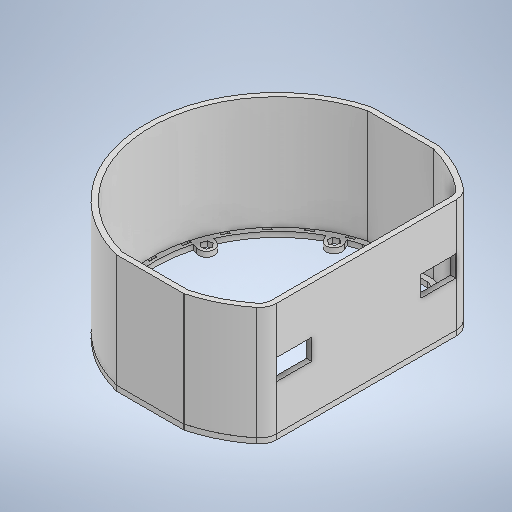
# Autodesk Inventor part: carcasa
Saved by Autodesk Inventor 2025.2 (Build 292293000, 293)
## iProperties
Created: 2025-08-27
Part Number: carcasa
Material: Generic
Document SubType Name: Modeling
Designer: cdavi
Density: 1 g/cm^3
Appearance: Default
Author: cdavi
Autodesk Inventor part; units mm, degrees
ref_plane "YZ Plane" through (0, 0, 0) normal (1, 0, 0) x (0, 1, 0)
ref_plane "XZ Plane" through (0, 0, 0) normal (0, 1, 0) x (-1, 0, 0)
ref_plane "XY Plane" through (0, 0, 0) normal (0, 0, 1) x (1, 0, 0)
sketch "Sketch1" plane through (0, 0, 0) normal (0, 1, 0) x (-1, 0, 0)
  line L0 (18.2688, 67.5) -> (-18.2688, 67.5)
  line L1 (0, 0) -> (-51, 0) construction
  line L2 (19.0722, 73.5) -> (-19.0722, 73.5)
  line L3 (18.2688, -67.5) -> (-18.5405, -67.5)
  line L4 (19.0722, -73.5) -> (-19.0722, -73.5)
  line L5 (0, 0) -> (0, 73.5) construction
  line L6 (-45, 48.734) -> (-45, -48.734)
  line L7 (-51, 51.7204) -> (-51, -51.7204)
  arc A0 (-40.8333, -56.8563) -> (-18.5405, -67.5) centre (0, 0) ccw
  arc A1 (-47.2121, -59.5568) -> (-19.5877, -73.4324) centre (0, 0) ccw
  arc A2 (19.5877, -73.4324) -> (19.5877, 73.4324) centre (0, 0) ccw
  arc A3 (-19.5877, 73.4324) -> (-47.2121, 59.5568) centre (0, 0) ccw
  arc A4 (18.8061, -67.4265) -> (18.8061, 67.4265) centre (0, 0) ccw
  arc A5 (-18.8061, 67.4265) -> (-40.8333, 56.8563) centre (0, 0) ccw
  arc A6 (-19.5877, -73.4324) -> (-19.0722, -73.5) centre (-19.0722, -71.5) ccw
  arc A7 (19.0722, -73.5) -> (19.5877, -73.4324) centre (19.0722, -71.5) ccw
  arc A8 (18.2688, -67.5) -> (18.8061, -67.4265) centre (18.2688, -65.5) ccw
  arc A9 (18.8061, 67.4265) -> (18.2688, 67.5) centre (18.2688, 65.5) ccw
  arc A10 (19.5877, 73.4324) -> (19.0722, 73.5) centre (19.0722, 71.5) ccw
  arc A11 (-18.2688, 67.5) -> (-18.8061, 67.4265) centre (-18.2688, 65.5) ccw
  arc A12 (-19.0722, 73.5) -> (-19.5877, 73.4324) centre (-19.0722, 71.5) ccw
  arc A13 (-40.8333, 56.8563) -> (-45, 48.734) centre (-35, 48.734) ccw
  arc A14 (-47.2121, 59.5568) -> (-51, 51.7204) centre (-41, 51.7204) ccw
  arc A15 (-51, -51.7204) -> (-47.2121, -59.5568) centre (-41, -51.7204) ccw
  arc A16 (-45, -48.734) -> (-40.8333, -56.8563) centre (-35, -48.734) ccw
  line L8 (18.9407, 70.5) -> (-18.9407, 70.5)
  arc A17 (-18.9407, 70.5) -> (-45.3485, 57.2059) centre (0, 0) ccw
  arc A18 (-45.3485, 57.2059) -> (-48, 51.7204) centre (-41, 51.7204) ccw
  line L9 (-48, 51.7204) -> (-48, -51.7204)
  arc A19 (-48, -51.7204) -> (-45.3485, -57.2059) centre (-41, -51.7204) ccw
  arc A20 (-45.3485, -57.2059) -> (-18.9407, -70.5) centre (0, 0) ccw
  line L10 (-18.9407, -70.5) -> (18.9407, -70.5)
  arc A21 (18.9407, -70.5) -> (18.9407, 70.5) centre (0, 0) ccw
  line L11 (18.9407, 70.5) -> (0, 0) construction
  line L12 (0, 0) -> (18.9407, -70.5) construction
  line L13 (0, 0) -> (-18.9407, -70.5) construction
  point P0 (-19.3326, 73.5)
  point P1 (18.5405, -67.5)
  point P2 (19.3326, -73.5)
  point P3 (-19.3326, -73.5)
  point P4 (-51, -56.3471)
  point P5 (-45, 53.619)
  point P6 (-45, -53.619)
  point P7 (-51, 56.3471)
  point P8 (19.3326, 73.5)
  point P9 (18.5405, 67.5)
  point P10 (-18.5405, 67.5)
  dimension "d2" = 67.5
  dimension "d4" = 6
  dimension "d6" = 45
  dimension "d7" = 6
  dimension "d8" = 2
  dimension "d9" = 10
  dimension "d10" = 70
  dimension "d11" = 76
  dimension "d12" = 70
  dimension "d13" = 76
  dimension "d185" = 3
  constraints: 55 point on circle, 28 end point, 22 centre point, 22 tangent, 11 point on line, 9 equal radius, 4 symmetric about line, 3 vertical, 2 coincident, 2 horizontal, 2 midpoint, 1 parallel, 7 other
  measures "d2" distance between parallel lines of L1 L0
  measures "d4" distance between parallel lines of L0 L2
  measures "d6" distance between parallel lines of L6 L5
  measures "d7" distance between parallel lines of L7 L6
  measures "d8" radius of A6
  measures "d9" radius of A13
  measures "d10" radius of A4
  measures "d11" radius of A2
  measures "d12" radius of A0
  measures "d13" radius of A1
  measures "d185" radial gap between concentric circles of A2 A21
extrude "Extrusion1" add sketch "Sketch1" along normal blind 65 contours A10 A2 A7 L4 A6 A1 A15 L7 A14 A3 A12 L2
sketch "Sketch2" plane through (51, 0, 51.7204) normal (1, 0, 0) x (0, 0, -1)
  line L0 (51.7204, 0) -> (51.7204, 67.372) construction
  line L1 (0.288, 38) -> (20.288, 38)
  line L2 (20.288, 38) -> (20.288, 26)
  line L3 (20.288, 26) -> (0.288, 26)
  line L4 (0.288, 26) -> (0.288, 38)
  line L5 (0, 0) -> (103.4408, 0) projected
  line L6 (-21.712, 0) -> (-21.712, 65) projected
  line L7 (103.1528, 38) -> (83.1528, 38)
  line L8 (83.1528, 38) -> (83.1528, 26)
  line L9 (83.1528, 26) -> (103.1528, 26)
  line L10 (103.1528, 26) -> (103.1528, 38)
  dimension "d16" = 26
  dimension "d17" = 22
  dimension "d18" = 12
  dimension "d19" = 20
  constraints: 18 end point, 4 symmetric about line, 2 parallel, 1 horizontal, 1 perpendicular, 1 vertical
  measures "d16" distance between parallel lines of L5 L3
  measures "d17" distance between parallel lines of L4 L6
  measures "d18" distance of L1.end L2.end
  measures "d19" distance of L1.start L1.end
extrude "Extrusion2" cut sketch "Sketch2" against normal blind 7
extrude "Extrusion4" add sketch "Sketch1" along normal blind 3 from surface at 65 separate body contours A9 A4 A8 L3 A0 A16 L6 A13 A5 A11 L0 | A10 A2 A7 L4 A6 A1 A15 L7 A14 A3 A12 L2 | A21 L10 A20 A19 L9 A18 A17 L8
sketch "Sketch5" plane through (-19.0722, 68, 73.5) normal (0, 1, 0) x (1, 0, 0)
  circle A0 centre (19.0722, 73.5) radius 8.5
  circle A1 centre (-10.9278, 73.5) radius 2.5
  line L0 (27.1963, 71) -> (36.0722, 71)
  line L1 (36.0722, 71) -> (36.0722, 76)
  line L2 (36.0722, 76) -> (27.1963, 76)
  point P0 (36.0722, 73.5)
  dimension "d26" = 17
  dimension "d27" = 5
  dimension "d31" = 5
  dimension "d32" = 17
  dimension "d47" = 30
  constraints: 6 end point, 2 centre point, 2 horizontal alignment, 2 perpendicular, 2 point on circle, 1 coincident, 1 horizontal, 1 midpoint
  measures "d26" diameter of A0
  measures "d27" diameter of A1
  measures "d31" distance between parallel lines of L2 L0
  measures "d32" distance from line of A0.centre L1
  measures "d47" distance of A0.centre A1.centre
extrude "Extrusion5" cut sketch "Sketch5" against normal through all bodies 2
sketch "Sketch6" plane through (0, 0, 0) normal (0, 1, 0) x (-1, 0, 0)
  circle A0 centre (0, 0) radius 67 construction
  line L0 (19.0722, 73.5) -> (-19.0722, 73.5) projected
  arc A1 (-19.5877, 73.4324) -> (-47.2121, 59.5568) centre (0, 0) ccw projected
  arc A2 (-47.2121, 59.5568) -> (-51, 51.7204) centre (-41, 51.7204) ccw projected
  line L1 (-51, 51.7204) -> (-51, -51.7204) projected
  arc A3 (-51, -51.7204) -> (-47.2121, -59.5568) centre (-41, -51.7204) ccw projected
  arc A4 (-47.2121, -59.5568) -> (-19.5877, -73.4324) centre (0, 0) ccw projected
  line L2 (-19.0722, -73.5) -> (19.0722, -73.5) projected
  arc A5 (19.5877, -73.4324) -> (19.5877, 73.4324) centre (0, 0) ccw projected
  line L3 (0, 0) -> (63.1919, 22.2662) construction
  line L4 (0, 0) -> (76, 0) construction
  circle A6 centre (63.1919, 22.2662) radius 2.95 construction
  line L5 (0, 0) -> (0, -67) construction
  circle A7 centre (28.3154, 60.7226) radius 2.95 construction
  line L6 (28.3154, 60.7226) -> (0, 0) construction
  circle A8 centre (-41.5, 20) radius 2.95 construction
  circle A9 centre (-28.3154, 60.7226) radius 2.95 construction
  line L7 (-28.3154, 60.7226) -> (0, 0) construction
  arc A10 (-19.5877, -73.4324) -> (-19.0722, -73.5) centre (-19.0722, -71.5) ccw projected
  arc A11 (19.0722, -73.5) -> (19.5877, -73.4324) centre (19.0722, -71.5) ccw projected
  arc A12 (19.5877, 73.4324) -> (19.0722, 73.5) centre (19.0722, 71.5) ccw projected
  arc A13 (-19.0722, 73.5) -> (-19.5877, 73.4324) centre (-19.0722, 71.5) ccw projected
  circle A14 centre (63.1919, -22.2662) radius 2.95 construction
  circle A15 centre (28.3154, -60.7226) radius 2.95 construction
  circle A16 centre (-41.5, -20) radius 2.95 construction
  circle A17 centre (-28.3154, -60.7226) radius 2.95 construction
  arc A18 (61.5547, 26.4578) -> (64.544, 17.9741) centre (63.1919, 22.2662) ccw
  arc A19 (24.1755, 62.4864) -> (32.3276, 58.685) centre (28.3154, 60.7226) ccw
  line L8 (60.2922, 22.8083) -> (62.2115, 25.0485)
  line L9 (62.2115, 25.0485) -> (65.1113, 24.5064)
  line L10 (65.1113, 24.5064) -> (66.0917, 21.724)
  line L11 (66.0917, 21.724) -> (64.1723, 19.4838)
  line L12 (64.1723, 19.4838) -> (61.2725, 20.026)
  line L13 (61.2725, 20.026) -> (60.2922, 22.8083)
  line L14 (25.8989, 59.0306) -> (25.6418, 61.9693)
  line L15 (25.6418, 61.9693) -> (28.0583, 63.6614)
  line L16 (28.0583, 63.6614) -> (30.7319, 62.4147)
  line L17 (30.7319, 62.4147) -> (30.989, 59.4759)
  line L18 (30.989, 59.4759) -> (28.5725, 57.7838)
  line L19 (28.5725, 57.7838) -> (25.8989, 59.0306)
  arc A20 (-41.5, 15.5) -> (-41.5, 24.5) centre (-41.5, 20) ccw
  line L20 (-44.0548, 18.525) -> (-44.0548, 21.475)
  line L21 (-44.0548, 21.475) -> (-41.5, 22.95)
  line L22 (-41.5, 22.95) -> (-38.9452, 21.475)
  line L23 (-38.9452, 21.475) -> (-38.9452, 18.525)
  line L24 (-38.9452, 18.525) -> (-41.5, 17.05)
  line L25 (-41.5, 17.05) -> (-44.0548, 18.525)
  line L26 (-41.5, 24.5) -> (-45, 24.5)
  line L27 (-41.5, 15.5) -> (-45, 15.5)
  arc A21 (-32.3276, 58.685) -> (-24.1755, 62.4864) centre (-28.3154, 60.7226) ccw
  line L28 (-28.5725, 57.7838) -> (-30.989, 59.4759)
  line L29 (-30.989, 59.4759) -> (-30.7319, 62.4147)
  line L30 (-30.7319, 62.4147) -> (-28.0583, 63.6614)
  line L31 (-28.0583, 63.6614) -> (-25.6418, 61.9693)
  line L32 (-25.6418, 61.9693) -> (-25.8989, 59.0306)
  line L33 (-25.8989, 59.0306) -> (-28.5725, 57.7838)
  line L34 (-32.3276, 58.685) -> (-33.6868, 61.3612)
  arc A22 (64.544, -17.9741) -> (61.5547, -26.4578) centre (63.1919, -22.2662) ccw
  arc A23 (32.3276, -58.685) -> (24.1755, -62.4864) centre (28.3154, -60.7226) ccw
  arc A24 (-41.5, -24.5) -> (-41.5, -15.5) centre (-41.5, -20) ccw
  line L35 (-41.5, -24.5) -> (-45, -24.5)
  line L36 (-41.5, -15.5) -> (-45, -15.5)
  arc A25 (-24.1755, -62.4864) -> (-32.3276, -58.685) centre (-28.3154, -60.7226) ccw
  line L37 (-32.3276, -58.685) -> (-33.6868, -61.3612)
  line L38 (60.2922, -22.8083) -> (62.2115, -25.0485)
  line L39 (62.2115, -25.0485) -> (65.1113, -24.5064)
  line L40 (65.1113, -24.5064) -> (66.0917, -21.724)
  line L41 (66.0917, -21.724) -> (64.1723, -19.4838)
  line L42 (64.1723, -19.4838) -> (61.2725, -20.026)
  line L43 (61.2725, -20.026) -> (60.2922, -22.8083)
  line L44 (25.8989, -59.0306) -> (25.6418, -61.9693)
  line L45 (25.6418, -61.9693) -> (28.0583, -63.6614)
  line L46 (28.0583, -63.6614) -> (30.7319, -62.4147)
  line L47 (30.7319, -62.4147) -> (30.989, -59.4759)
  line L48 (30.989, -59.4759) -> (28.5725, -57.7838)
  line L49 (28.5725, -57.7838) -> (25.8989, -59.0306)
  line L50 (-28.5725, -57.7838) -> (-30.989, -59.4759)
  line L51 (-30.989, -59.4759) -> (-30.7319, -62.4147)
  line L52 (-30.7319, -62.4147) -> (-28.0583, -63.6614)
  line L53 (-28.0583, -63.6614) -> (-25.6418, -61.9693)
  line L54 (-25.6418, -61.9693) -> (-25.8989, -59.0306)
  line L55 (-25.8989, -59.0306) -> (-28.5725, -57.7838)
  line L56 (-44.0548, -18.525) -> (-44.0548, -21.475)
  line L57 (-44.0548, -21.475) -> (-41.5, -22.95)
  line L58 (-41.5, -22.95) -> (-38.9452, -21.475)
  line L59 (-38.9452, -21.475) -> (-38.9452, -18.525)
  line L60 (-38.9452, -18.525) -> (-41.5, -17.05)
  line L61 (-41.5, -17.05) -> (-44.0548, -18.525)
  line L62 (61.5547, 26.4578) -> (64.3507, 27.5498)
  line L63 (64.544, 17.9741) -> (67.4069, 18.876)
  line L64 (32.3276, 58.685) -> (33.6868, 61.3612)
  line L65 (61.5547, -26.4578) -> (64.3507, -27.5498)
  line L66 (64.544, -17.9741) -> (67.4069, -18.876)
  line L67 (32.3276, -58.685) -> (33.6868, -61.3612)
  line L68 (-24.1755, 62.4864) -> (-25.3519, 65.2478)
  line L69 (24.1755, 62.4864) -> (25.3519, 65.2478)
  line L70 (-24.1755, -62.4864) -> (-25.3519, -65.2478)
  line L71 (24.1755, -62.4864) -> (25.3519, -65.2478)
  arc A26 (-18.5405, 67.5) -> (-43.4848, 54.855) centre (0, 0) ccw
  line L72 (-18.5405, 67.5) -> (18.5405, 67.5)
  arc A27 (18.5405, -67.5) -> (18.5405, 67.5) centre (0, 0) ccw
  line L73 (18.5405, -67.5) -> (-18.5405, -67.5)
  arc A28 (-43.4848, -54.855) -> (-18.5405, -67.5) centre (0, 0) ccw
  arc A29 (-45, -51.7204) -> (-43.4848, -54.855) centre (-41, -51.7204) ccw
  line L74 (-45, -51.7204) -> (-45, 51.7204)
  arc A30 (-43.4848, 54.855) -> (-45, 51.7204) centre (-41, 51.7204) ccw
  point P0 (28.3154, 60.7226)
  point P1 (28.3154, 60.7226)
  point P2 (61.5547, -26.4578)
  point P3 (32.3276, -58.685)
  point P4 (-24.1755, -62.4864)
  dimension "d33" = 134
  dimension "d39" = 5.9
  dimension "d37" = 19.41
  dimension "d38" = 25
  dimension "d40" = 20
  dimension "d42" = 25
  dimension "d61" = 9
  dimension "d62" = 9
  dimension "d63" = 9
  dimension "d64" = 9
  dimension "d186" = 6
  dimension "d187" = 3.5
  constraints: 144 end point, 48 symmetric about line, 27 point on circle, 17 centre point, 10 coincident, 8 tangent, 4 perpendicular, 3 horizontal, 2 point on line, 1 vertical, 93 other
  measures "d37" angle of L4 L3
  measures "d38" angle of L5 L6
  measures "d40" distance from line of point (-41.5, 20) L4
  measures "d42" angle of L5 L7
  measures "d61" diameter of A18
  measures "d62" diameter of A19
  measures "d63" diameter of A20
  measures "d64" diameter of A21
  measures "d186" radial gap between concentric circles of A1 A26
  measures "d187" distance from line of L74 A20.centre
extrude "Extrusion6" add sketch "Sketch6" against normal blind 3 separate body contours A12 A5 A11 L2 A10 A4 A3 L1 A2 A1 A13 L0 | L62 A27 L63 A18 | L64 A19 L69 A27 | A27 L65 A22 L66 | A27 L71 A23 L67 | L68 A21 L34 A26 | A28 L37 A25 L70 | L26 A20 L27 L74 | L36 A24 L35 L74
sketch "Sketch8" plane through (0, 0, 0) normal (0, 1, 0) x (1, 0, 0)
  arc A0 (-19.5877, 73.4324) -> (-19.5877, -73.4324) centre (0, 0) ccw projected
  line L0 (-76, 0) -> (-70, 0)
  line L1 (-73, 0) -> (-73, -2)
  line L2 (-73, 0) -> (-73, 2)
  line L3 (-73, 2) -> (-71.5, 2)
  line L4 (-71.5, 2) -> (-71.5, -2)
  line L5 (-71.5, -2) -> (-74.5, -2)
  line L6 (-74.5, -2) -> (-74.5, 2)
  line L7 (-74.5, 2) -> (-71.5, 2)
  line L8 (-69.901, -15.1692) -> (-68.9437, -19.053)
  line L9 (-68.9437, -19.053) -> (-71.8565, -19.7709)
  line L10 (-71.8565, -19.7709) -> (-72.8138, -15.8871)
  line L11 (-71.3574, -15.5282) -> (-69.901, -15.1692)
  line L12 (-72.8138, -15.8871) -> (-69.901, -15.1692)
  line L13 (-64.2396, -31.4568) -> (-62.3807, -34.9986)
  line L14 (-62.3807, -34.9986) -> (-65.037, -36.3928)
  line L15 (-65.037, -36.3928) -> (-66.8959, -32.851)
  line L16 (-65.5677, -32.1539) -> (-64.2396, -31.4568)
  line L17 (-66.8959, -32.851) -> (-64.2396, -31.4568)
  line L18 (-54.8448, -45.9162) -> (-52.1923, -48.9103)
  line L19 (-52.1923, -48.9103) -> (-54.4378, -50.8997)
  line L20 (-54.4378, -50.8997) -> (-57.0903, -47.9056)
  line L21 (-55.9675, -46.9109) -> (-54.8448, -45.9162)
  line L22 (-57.0903, -47.9056) -> (-54.8448, -45.9162)
  line L23 (-42.2626, -57.7072) -> (-38.9707, -59.9795)
  line L24 (-38.9707, -59.9795) -> (-40.6749, -62.4484)
  line L25 (-40.6749, -62.4484) -> (-43.9668, -60.1762)
  line L26 (-43.1147, -58.9417) -> (-42.2626, -57.7072)
  line L27 (-43.9668, -60.1762) -> (-42.2626, -57.7072)
  line L28 (-27.2243, -66.1445) -> (-23.4842, -67.5629)
  line L29 (-23.4842, -67.5629) -> (-24.548, -70.3679)
  line L30 (-24.548, -70.3679) -> (-28.2881, -68.9495)
  line L31 (-27.7562, -67.547) -> (-27.2243, -66.1445)
  line L32 (-28.2881, -68.9495) -> (-27.2243, -66.1445)
  line L33 (-10.6038, -70.7376) -> (-6.633, -71.2198)
  line L34 (-6.633, -71.2198) -> (-6.9946, -74.1979)
  line L35 (-6.9946, -74.1979) -> (-10.9654, -73.7157)
  line L36 (-10.7846, -72.2267) -> (-10.6038, -70.7376)
  line L37 (-10.9654, -73.7157) -> (-10.6038, -70.7376)
  line L38 (6.633, -71.2198) -> (10.6038, -70.7376)
  line L39 (10.6038, -70.7376) -> (10.9654, -73.7157)
  line L40 (10.9654, -73.7157) -> (6.9946, -74.1979)
  line L41 (6.8138, -72.7088) -> (6.633, -71.2198)
  line L42 (6.9946, -74.1979) -> (6.633, -71.2198)
  line L43 (23.4842, -67.5629) -> (27.2243, -66.1445)
  line L44 (27.2243, -66.1445) -> (28.2881, -68.9495)
  line L45 (28.2881, -68.9495) -> (24.548, -70.3679)
  line L46 (24.0161, -68.9654) -> (23.4842, -67.5629)
  line L47 (24.548, -70.3679) -> (23.4842, -67.5629)
  line L48 (38.9707, -59.9795) -> (42.2626, -57.7072)
  line L49 (42.2626, -57.7072) -> (43.9668, -60.1762)
  line L50 (43.9668, -60.1762) -> (40.6749, -62.4484)
  line L51 (39.8228, -61.214) -> (38.9707, -59.9795)
  line L52 (40.6749, -62.4484) -> (38.9707, -59.9795)
  line L53 (52.1923, -48.9103) -> (54.8448, -45.9162)
  line L54 (54.8448, -45.9162) -> (57.0903, -47.9056)
  line L55 (57.0903, -47.9056) -> (54.4378, -50.8997)
  line L56 (53.315, -49.905) -> (52.1923, -48.9103)
  line L57 (54.4378, -50.8997) -> (52.1923, -48.9103)
  line L58 (62.3807, -34.9986) -> (64.2396, -31.4568)
  line L59 (64.2396, -31.4568) -> (66.8959, -32.851)
  line L60 (66.8959, -32.851) -> (65.037, -36.3928)
  line L61 (63.7088, -35.6957) -> (62.3807, -34.9986)
  line L62 (65.037, -36.3928) -> (62.3807, -34.9986)
  line L63 (68.9437, -19.053) -> (69.901, -15.1692)
  line L64 (69.901, -15.1692) -> (72.8138, -15.8871)
  line L65 (72.8138, -15.8871) -> (71.8565, -19.7709)
  line L66 (70.4001, -19.4119) -> (68.9437, -19.053)
  line L67 (71.8565, -19.7709) -> (68.9437, -19.053)
  line L68 (71.5, -2) -> (71.5, 2)
  line L69 (71.5, 2) -> (74.5, 2)
  line L70 (74.5, 2) -> (74.5, -2)
  line L71 (73, -2) -> (71.5, -2)
  line L72 (74.5, -2) -> (71.5, -2)
  line L73 (69.901, 15.1692) -> (68.9437, 19.053)
  line L74 (68.9437, 19.053) -> (71.8565, 19.7709)
  line L75 (71.8565, 19.7709) -> (72.8138, 15.8871)
  line L76 (71.3574, 15.5282) -> (69.901, 15.1692)
  line L77 (72.8138, 15.8871) -> (69.901, 15.1692)
  line L78 (64.2396, 31.4568) -> (62.3807, 34.9986)
  line L79 (62.3807, 34.9986) -> (65.037, 36.3928)
  line L80 (65.037, 36.3928) -> (66.8959, 32.851)
  line L81 (65.5677, 32.1539) -> (64.2396, 31.4568)
  line L82 (66.8959, 32.851) -> (64.2396, 31.4568)
  line L83 (54.8448, 45.9162) -> (52.1923, 48.9103)
  line L84 (52.1923, 48.9103) -> (54.4378, 50.8997)
  line L85 (54.4378, 50.8997) -> (57.0903, 47.9056)
  line L86 (55.9675, 46.9109) -> (54.8448, 45.9162)
  line L87 (57.0903, 47.9056) -> (54.8448, 45.9162)
  line L88 (42.2626, 57.7072) -> (38.9707, 59.9795)
  line L89 (38.9707, 59.9795) -> (40.6749, 62.4484)
  line L90 (40.6749, 62.4484) -> (43.9668, 60.1762)
  line L91 (43.1147, 58.9417) -> (42.2626, 57.7072)
  line L92 (43.9668, 60.1762) -> (42.2626, 57.7072)
  line L93 (27.2243, 66.1445) -> (23.4842, 67.5629)
  line L94 (23.4842, 67.5629) -> (24.548, 70.3679)
  line L95 (24.548, 70.3679) -> (28.2881, 68.9495)
  line L96 (27.7562, 67.547) -> (27.2243, 66.1445)
  line L97 (28.2881, 68.9495) -> (27.2243, 66.1445)
  line L98 (10.6038, 70.7376) -> (6.633, 71.2198)
  line L99 (6.633, 71.2198) -> (6.9946, 74.1979)
  line L100 (6.9946, 74.1979) -> (10.9654, 73.7157)
  line L101 (10.7846, 72.2267) -> (10.6038, 70.7376)
  line L102 (10.9654, 73.7157) -> (10.6038, 70.7376)
  line L103 (-6.633, 71.2198) -> (-10.6038, 70.7376)
  line L104 (-10.6038, 70.7376) -> (-10.9654, 73.7157)
  line L105 (-10.9654, 73.7157) -> (-6.9946, 74.1979)
  line L106 (-6.8138, 72.7088) -> (-6.633, 71.2198)
  line L107 (-6.9946, 74.1979) -> (-6.633, 71.2198)
  line L108 (-23.4842, 67.5629) -> (-27.2243, 66.1445)
  line L109 (-27.2243, 66.1445) -> (-28.2881, 68.9495)
  line L110 (-28.2881, 68.9495) -> (-24.548, 70.3679)
  line L111 (-24.0161, 68.9654) -> (-23.4842, 67.5629)
  line L112 (-24.548, 70.3679) -> (-23.4842, 67.5629)
  line L113 (-38.9707, 59.9795) -> (-42.2626, 57.7072)
  line L114 (-42.2626, 57.7072) -> (-43.9668, 60.1762)
  line L115 (-43.9668, 60.1762) -> (-40.6749, 62.4484)
  line L116 (-39.8228, 61.214) -> (-38.9707, 59.9795)
  line L117 (-40.6749, 62.4484) -> (-38.9707, 59.9795)
  line L118 (-52.1923, 48.9103) -> (-54.8448, 45.9162)
  line L119 (-54.8448, 45.9162) -> (-57.0903, 47.9056)
  line L120 (-57.0903, 47.9056) -> (-54.4378, 50.8997)
  line L121 (-53.315, 49.905) -> (-52.1923, 48.9103)
  line L122 (-54.4378, 50.8997) -> (-52.1923, 48.9103)
  line L123 (-62.3807, 34.9986) -> (-64.2396, 31.4568)
  line L124 (-64.2396, 31.4568) -> (-66.8959, 32.851)
  line L125 (-66.8959, 32.851) -> (-65.037, 36.3928)
  line L126 (-63.7088, 35.6957) -> (-62.3807, 34.9986)
  line L127 (-65.037, 36.3928) -> (-62.3807, 34.9986)
  line L128 (-68.9437, 19.053) -> (-69.901, 15.1692)
  line L129 (-69.901, 15.1692) -> (-72.8138, 15.8871)
  line L130 (-72.8138, 15.8871) -> (-71.8565, 19.7709)
  line L131 (-70.4001, 19.4119) -> (-68.9437, 19.053)
  line L132 (-71.8565, 19.7709) -> (-68.9437, 19.053)
  arc A1 (-67.4069, 18.876) -> (-67.4069, -18.876) centre (0, 0) ccw projected
  point P0 (-73, 2)
  dimension "d132" = 2
  dimension "d133" = 2
  dimension "d134" = 1.5
  dimension "d135" = 4
  dimension "d136" = 3
  dimension "d137" = 4
  dimension "d140" = 360
  dimension "d205" = 71.5
  constraints: 266 end point, 26 point on line, 3 perpendicular, 2 vertical, 1 horizontal, 1 horizontal alignment, 1 midpoint, 1 point on circle, 261 other
  measures "d132" distance of L1.start L1.end
  measures "d133" distance of L1.start L2.end
  measures "d134" distance of L2.end L3.end
  measures "d135" distance of L3.end L4.end
  measures "d136" distance of L4.end L5.end
  measures "d137" distance of L5.end L6.end
  measures "d205" distance from line of L4 A1.centre
extrude "Extrusion7" cut sketch "Sketch8" against normal blind 20.75 contours L6 L7 L2 L0 | L0 L1 L5 L6 | L2 L3 L4 L0 | L0 L4 L5 L1 | L8 L9 L10 L12 L11 | L13 L14 L15 L17 L16 | L18 L19 L20 L22 L21 | L23 L24 L25 L27 L26 | L28 L29 L30 L32 L31 | L108 L109 L110 L112 L111 | L113 L114 L115 L117 L116 | L118 L119 L120 L122 L121 | L123 L124 L125 L127 L126 | L128 L129 L130 L132 L131 bodies 3
sketch "Sketch9" plane through (0, 0, 0) normal (0, 1, 0) x (1, 0, 0)
  line L0 (19.0722, -73.5) -> (-19.0722, -73.5) projected
  line L1 (-18.5405, -67.5) -> (-18.5405, -73.5)
  line L2 (18.5405, -67.5) -> (18.5405, -73.5)
  line L3 (-18.5405, -70.5) -> (18.5405, -70.5)
  line L4 (0, -70.5) -> (0, -73.5)
  line L5 (0, -70.5) -> (0, -67.4265)
  line L6 (0, -70.5) -> (18.5405, -70.5)
  line L7 (9.2702, -70.5) -> (7.2702, -70.5)
  line L8 (7.2702, -70.5) -> (7.2702, -69.15)
  line L9 (7.2702, -69.15) -> (11.2702, -69.15)
  line L10 (11.2702, -69.15) -> (11.2702, -71.85)
  line L11 (11.2702, -71.85) -> (7.2702, -71.85)
  line L12 (7.2702, -71.85) -> (7.2702, -70.5)
  line L13 (-7.2702, -70.5) -> (-7.2702, -69.15)
  line L14 (-7.2702, -69.15) -> (-11.2702, -69.15)
  line L15 (-11.2702, -69.15) -> (-11.2702, -71.85)
  line L16 (-11.2702, -71.85) -> (-7.2702, -71.85)
  line L17 (-7.2702, -71.85) -> (-7.2702, -70.5)
  arc A0 (-19.5877, 73.4324) -> (-19.5877, -73.4324) centre (0, 0) ccw projected
  line L18 (-76, 0) -> (51, 0)
  line L19 (51, 51.7204) -> (51, -51.7204) projected
  line L20 (7.2702, 70.5) -> (7.2702, 69.15)
  line L21 (7.2702, 69.15) -> (11.2702, 69.15)
  line L22 (11.2702, 69.15) -> (11.2702, 71.85)
  line L23 (11.2702, 71.85) -> (7.2702, 71.85)
  line L24 (7.2702, 71.85) -> (7.2702, 70.5)
  line L25 (-7.2702, 69.15) -> (-11.2702, 69.15)
  line L26 (-11.2702, 69.15) -> (-11.2702, 71.85)
  line L27 (-11.2702, 71.85) -> (-7.2702, 71.85)
  line L28 (-7.2702, 71.85) -> (-7.2702, 70.5)
  line L29 (-7.2702, 70.5) -> (-7.2702, 69.15)
  line L30 (11.2702, -70.5) -> (11.2702, -71.85)
  line L31 (7.2702, -71.85) -> (7.2702, -70.5)
  line L32 (7.2702, -69.15) -> (7.2702, -70.5)
  line L33 (7.2702, -69.15) -> (11.2702, -69.15)
  line L34 (11.2702, -71.85) -> (7.2702, -71.85)
  dimension "d144" = 2
  dimension "d145" = 1.35
  dimension "d146" = 4
  dimension "d147" = 2.7
  dimension "d148" = 4
  constraints: 66 end point, 15 symmetric about line, 8 perpendicular, 7 midpoint, 7 point on line, 2 collinear, 2 vertical, 1 coincident, 1 horizontal, 1 point on circle, 1 vertical alignment
  measures "d144" distance of L7.start L7.end
  measures "d145" distance of L7.end L8.end
  measures "d146" distance of L8.end L9.end
  measures "d147" distance of L9.end L10.end
  measures "d148" distance of L10.end L11.end
extrude "Extrusion8" cut sketch "Sketch9" against normal blind 49.25 contours L10 L11 L12 L3 | L3 L8 L9 L10 | L17 L16 L15 L3 | L3 L15 L14 L13 | L24 L23 L22 L21 L20 | L25 L26 L27 L28 L29 bodies 3
sketch "Sketch10" plane through (0, 0, 0) normal (0, 1, 0) x (1, 0, 0)
  line L0 (45, 49) -> (51, 49)
  line L1 (51, 51.7204) -> (51, -51.7204) projected
  line L2 (48, 49) -> (48, -49)
  line L3 (45, -49) -> (51, -49)
  line L4 (48, 0) -> (48, -49)
  line L5 (48, -24.5) -> (48, -12.3165)
  line L6 (48, -12.3165) -> (48, -10.3165)
  line L7 (48, -10.3165) -> (49.35, -10.3165)
  line L8 (48, -12.3165) -> (48, -14.3165)
  line L9 (48, -14.3165) -> (46.65, -14.3165)
  line L10 (46.65, -14.3165) -> (49.35, -14.3165)
  line L11 (49.35, -14.3165) -> (49.35, -10.3165)
  line L12 (49.35, -10.3165) -> (46.65, -10.3165)
  line L13 (46.65, -10.3165) -> (46.65, -14.3165)
  line L14 (48, -24.5) -> (45, -24.5)
  line L15 (46.65, -34.6835) -> (49.35, -34.6835)
  line L16 (49.35, -34.6835) -> (49.35, -38.6835)
  line L17 (49.35, -38.6835) -> (46.65, -38.6835)
  line L18 (46.65, -38.6835) -> (46.65, -34.6835)
  line L19 (48, 0) -> (45, 0)
  line L20 (48, 10.3165) -> (49.35, 10.3165)
  line L21 (46.65, 14.3165) -> (49.35, 14.3165)
  line L22 (49.35, 14.3165) -> (49.35, 10.3165)
  line L23 (49.35, 10.3165) -> (46.65, 10.3165)
  line L24 (46.65, 10.3165) -> (46.65, 14.3165)
  line L25 (46.65, 34.6835) -> (49.35, 34.6835)
  line L26 (46.65, 38.6835) -> (46.65, 34.6835)
  line L27 (49.35, 38.6835) -> (46.65, 38.6835)
  line L28 (49.35, 34.6835) -> (49.35, 38.6835)
  line L29 (45, 51.7204) -> (45, 24.5) projected
  line L30 (45, -24.5) -> (45, -51.7204) projected
  line L31 (45, 15.5) -> (45, -15.5) projected
  point P0 (0, 0)
  point P1 (45, 0)
  dimension "d151" = 12.1835
  dimension "d152" = 2
  dimension "d153" = 1.35
  dimension "d154" = 2
  dimension "d155" = 1.35
  constraints: 56 end point, 13 symmetric about line, 7 point on line, 5 midpoint, 4 horizontal, 4 perpendicular, 2 horizontal alignment, 2 parallel, 2 vertical
  measures "d151" distance of L5.start L5.end
  measures "d152" distance of L5.end L6.end
  measures "d153" distance of L6.end L7.end
  measures "d154" distance of L5.end L8.end
  measures "d155" distance of L8.end L9.end
extrude "Extrusion9" cut sketch "Sketch10" against normal blind 52.5 contours L27 L28 L25 L2 | L2 L25 L26 L27 | L21 L22 L20 L2 | L2 L23 L24 L21 | L17 L18 L15 L2 | L2 L15 L16 L17 | L7 L11 L10 L2 | L2 L9 L13 L12 bodies 3
sketch "Sketch11" plane through (0, 0, 0) normal (0, 1, 0) x (1, 0, 0)
  line L0 (-18.8061, -67.4265) -> (18.8061, -67.4265) projected
  arc A0 (47.2121, -59.5568) -> (51, -51.7204) centre (41, -51.7204) ccw projected
  line L1 (-70, 0) -> (-76, 0)
  arc A1 (-19.5877, 73.4324) -> (-19.5877, -73.4324) centre (0, 0) ccw projected
  line L2 (-73, 0) -> (-73, -2)
  line L3 (-73, -2) -> (-71.5, -2)
  line L4 (-73, 0) -> (-73, 2)
  line L5 (-73, 2) -> (-74.5, 2)
  line L6 (-71.5, -2) -> (-74.5, -2)
  line L7 (-74.5, -2) -> (-74.5, 2)
  line L8 (-74.5, 2) -> (-71.5, 2)
  line L9 (-71.5, 2) -> (-71.5, -2)
  line L10 (-71.8565, -19.7709) -> (-72.8138, -15.8871)
  line L11 (-68.9437, -19.053) -> (-71.8565, -19.7709)
  line L12 (-69.901, -15.1692) -> (-68.9437, -19.053)
  line L13 (-72.8138, -15.8871) -> (-69.901, -15.1692)
  line L14 (-65.037, -36.3928) -> (-66.8959, -32.851)
  line L15 (-62.3807, -34.9986) -> (-65.037, -36.3928)
  line L16 (-64.2396, -31.4568) -> (-62.3807, -34.9986)
  line L17 (-66.8959, -32.851) -> (-64.2396, -31.4568)
  line L18 (-54.4378, -50.8997) -> (-57.0903, -47.9056)
  line L19 (-52.1923, -48.9103) -> (-54.4378, -50.8997)
  line L20 (-54.8448, -45.9162) -> (-52.1923, -48.9103)
  line L21 (-57.0903, -47.9056) -> (-54.8448, -45.9162)
  line L22 (-40.6749, -62.4484) -> (-43.9668, -60.1762)
  line L23 (-38.9707, -59.9795) -> (-40.6749, -62.4484)
  line L24 (-42.2626, -57.7072) -> (-38.9707, -59.9795)
  line L25 (-43.9668, -60.1762) -> (-42.2626, -57.7072)
  line L26 (-24.548, -70.3679) -> (-28.2881, -68.9495)
  line L27 (-23.4842, -67.5629) -> (-24.548, -70.3679)
  line L28 (-27.2243, -66.1445) -> (-23.4842, -67.5629)
  line L29 (-28.2881, -68.9495) -> (-27.2243, -66.1445)
  line L30 (-6.9946, -74.1979) -> (-10.9654, -73.7157)
  line L31 (-6.633, -71.2198) -> (-6.9946, -74.1979)
  line L32 (-10.6038, -70.7376) -> (-6.633, -71.2198)
  line L33 (-10.9654, -73.7157) -> (-10.6038, -70.7376)
  line L34 (10.9654, -73.7157) -> (6.9946, -74.1979)
  line L35 (10.6038, -70.7376) -> (10.9654, -73.7157)
  line L36 (6.633, -71.2198) -> (10.6038, -70.7376)
  line L37 (6.9946, -74.1979) -> (6.633, -71.2198)
  line L38 (28.2881, -68.9495) -> (24.548, -70.3679)
  line L39 (27.2243, -66.1445) -> (28.2881, -68.9495)
  line L40 (23.4842, -67.5629) -> (27.2243, -66.1445)
  line L41 (24.548, -70.3679) -> (23.4842, -67.5629)
  line L42 (43.9668, -60.1762) -> (40.6749, -62.4484)
  line L43 (42.2626, -57.7072) -> (43.9668, -60.1762)
  line L44 (38.9707, -59.9795) -> (42.2626, -57.7072)
  line L45 (40.6749, -62.4484) -> (38.9707, -59.9795)
  line L46 (57.0903, -47.9056) -> (54.4378, -50.8997)
  line L47 (54.8448, -45.9162) -> (57.0903, -47.9056)
  line L48 (52.1923, -48.9103) -> (54.8448, -45.9162)
  line L49 (54.4378, -50.8997) -> (52.1923, -48.9103)
  line L50 (66.8959, -32.851) -> (65.037, -36.3928)
  line L51 (64.2396, -31.4568) -> (66.8959, -32.851)
  line L52 (62.3807, -34.9986) -> (64.2396, -31.4568)
  line L53 (65.037, -36.3928) -> (62.3807, -34.9986)
  line L54 (72.8138, -15.8871) -> (71.8565, -19.7709)
  line L55 (69.901, -15.1692) -> (72.8138, -15.8871)
  line L56 (68.9437, -19.053) -> (69.901, -15.1692)
  line L57 (71.8565, -19.7709) -> (68.9437, -19.053)
  line L58 (74.5, 2) -> (74.5, -2)
  line L59 (71.5, 2) -> (74.5, 2)
  line L60 (71.5, -2) -> (71.5, 2)
  line L61 (74.5, -2) -> (71.5, -2)
  line L62 (71.8565, 19.7709) -> (72.8138, 15.8871)
  line L63 (68.9437, 19.053) -> (71.8565, 19.7709)
  line L64 (69.901, 15.1692) -> (68.9437, 19.053)
  line L65 (72.8138, 15.8871) -> (69.901, 15.1692)
  line L66 (65.037, 36.3928) -> (66.8959, 32.851)
  line L67 (62.3807, 34.9986) -> (65.037, 36.3928)
  line L68 (64.2396, 31.4568) -> (62.3807, 34.9986)
  line L69 (66.8959, 32.851) -> (64.2396, 31.4568)
  line L70 (54.4378, 50.8997) -> (57.0903, 47.9056)
  line L71 (52.1923, 48.9103) -> (54.4378, 50.8997)
  line L72 (54.8448, 45.9162) -> (52.1923, 48.9103)
  line L73 (57.0903, 47.9056) -> (54.8448, 45.9162)
  line L74 (40.6749, 62.4484) -> (43.9668, 60.1762)
  line L75 (38.9707, 59.9795) -> (40.6749, 62.4484)
  line L76 (42.2626, 57.7072) -> (38.9707, 59.9795)
  line L77 (43.9668, 60.1762) -> (42.2626, 57.7072)
  line L78 (24.548, 70.3679) -> (28.2881, 68.9495)
  line L79 (23.4842, 67.5629) -> (24.548, 70.3679)
  line L80 (27.2243, 66.1445) -> (23.4842, 67.5629)
  line L81 (28.2881, 68.9495) -> (27.2243, 66.1445)
  line L82 (6.9946, 74.1979) -> (10.9654, 73.7157)
  line L83 (6.633, 71.2198) -> (6.9946, 74.1979)
  line L84 (10.6038, 70.7376) -> (6.633, 71.2198)
  line L85 (10.9654, 73.7157) -> (10.6038, 70.7376)
  line L86 (-10.9654, 73.7157) -> (-6.9946, 74.1979)
  line L87 (-10.6038, 70.7376) -> (-10.9654, 73.7157)
  line L88 (-6.633, 71.2198) -> (-10.6038, 70.7376)
  line L89 (-6.9946, 74.1979) -> (-6.633, 71.2198)
  line L90 (-28.2881, 68.9495) -> (-24.548, 70.3679)
  line L91 (-27.2243, 66.1445) -> (-28.2881, 68.9495)
  line L92 (-23.4842, 67.5629) -> (-27.2243, 66.1445)
  line L93 (-24.548, 70.3679) -> (-23.4842, 67.5629)
  line L94 (-43.9668, 60.1762) -> (-40.6749, 62.4484)
  line L95 (-42.2626, 57.7072) -> (-43.9668, 60.1762)
  line L96 (-38.9707, 59.9795) -> (-42.2626, 57.7072)
  line L97 (-40.6749, 62.4484) -> (-38.9707, 59.9795)
  line L98 (-57.0903, 47.9056) -> (-54.4378, 50.8997)
  line L99 (-54.8448, 45.9162) -> (-57.0903, 47.9056)
  line L100 (-52.1923, 48.9103) -> (-54.8448, 45.9162)
  line L101 (-54.4378, 50.8997) -> (-52.1923, 48.9103)
  line L102 (-66.8959, 32.851) -> (-65.037, 36.3928)
  line L103 (-64.2396, 31.4568) -> (-66.8959, 32.851)
  line L104 (-62.3807, 34.9986) -> (-64.2396, 31.4568)
  line L105 (-65.037, 36.3928) -> (-62.3807, 34.9986)
  line L106 (-72.8138, 15.8871) -> (-71.8565, 19.7709)
  line L107 (-69.901, 15.1692) -> (-72.8138, 15.8871)
  line L108 (-68.9437, 19.053) -> (-69.901, 15.1692)
  line L109 (-71.8565, 19.7709) -> (-68.9437, 19.053)
  arc A2 (-67.4069, 18.876) -> (-67.4069, -18.876) centre (0, 0) ccw projected
  point P0 (19.5877, -73.4324)
  dimension "d158" = 6
  dimension "d159" = 2
  dimension "d160" = 1.5
  dimension "d161" = 2
  dimension "d162" = 1.5
  dimension "d165" = 360
  constraints: 218 end point, 3 perpendicular, 2 horizontal, 2 parallel, 2 vertical, 1 horizontal alignment, 1 midpoint, 1 point on circle, 209 other
  measures "d158" distance of L1.start L1.end
  measures "d159" distance of L2.start L2.end
  measures "d160" distance of L2.end L3.end
  measures "d161" distance of L2.start L4.end
  measures "d162" distance of L4.end L5.end
extrude "Extrusion10" cut sketch "Sketch11" against normal blind 38.5 contours L38 L41 L40 L39 | L42 L45 L44 L43 | L74 L77 L76 L75 | L78 L81 L80 L79 bodies 3
sketch "Sketch13" plane through (-19.0722, 68, 73.5) normal (0, 1, 0) x (1, 0, 0)
  line L0 (-55.4278, 71.5) -> (-52.4278, 71.5) projected
  line L1 (-55.4278, 75.5) -> (-55.4278, 71.5) projected
  line L2 (-52.4278, 75.5) -> (-55.4278, 75.5) projected
  line L3 (-52.4278, 71.5) -> (-52.4278, 75.5) projected
  line L4 (19.0722, 73.5) -> (-52.4278, 73.5)
  line L5 (-52.4278, 75.5) -> (-52.4278, 71.5)
  line L6 (-55.4278, 71.5) -> (-55.4278, 75.5)
  line L7 (-55.4278, 75.5) -> (-52.4278, 75.5)
  line L8 (-55.4278, 71.5) -> (-52.4278, 71.5)
  arc A0 (-0.5155, 146.9324) -> (-0.5155, 0.0676) centre (19.0722, 73.5) ccw projected
  arc A1 (27.1963, 76) -> (27.1963, 71) centre (19.0722, 73.5) ccw projected
  circle A2 centre (19.0722, 73.5) radius 76
  line L9 (-53.7416, 57.6129) -> (-50.8287, 58.3308)
  line L10 (-52.7843, 53.7291) -> (-53.7416, 57.6129)
  line L11 (-52.7843, 53.7291) -> (-49.8715, 54.447)
  line L12 (-50.8287, 58.3308) -> (-49.8715, 54.447)
  line L13 (-47.8237, 40.649) -> (-45.1673, 42.0432)
  line L14 (-45.9648, 37.1072) -> (-47.8237, 40.649)
  line L15 (-45.9648, 37.1072) -> (-43.3084, 38.5014)
  line L16 (-45.1673, 42.0432) -> (-43.3084, 38.5014)
  line L17 (-38.0181, 25.5944) -> (-35.7725, 27.5838)
  line L18 (-35.3656, 22.6003) -> (-38.0181, 25.5944)
  line L19 (-35.3656, 22.6003) -> (-33.12, 24.5897)
  line L20 (-35.7725, 27.5838) -> (-33.12, 24.5897)
  line L21 (-24.8946, 13.3238) -> (-23.1904, 15.7928)
  line L22 (-21.6026, 11.0516) -> (-24.8946, 13.3238)
  line L23 (-21.6026, 11.0516) -> (-19.8984, 13.5205)
  line L24 (-23.1904, 15.7928) -> (-19.8984, 13.5205)
  line L25 (-9.2159, 4.5505) -> (-8.1521, 7.3555)
  line L26 (-5.4758, 3.1321) -> (-9.2159, 4.5505)
  line L27 (-5.4758, 3.1321) -> (-4.412, 5.9371)
  line L28 (-8.1521, 7.3555) -> (-4.412, 5.9371)
  line L29 (8.1068, -0.2157) -> (8.4684, 2.7624)
  line L30 (12.0777, -0.6979) -> (8.1068, -0.2157)
  line L31 (12.0777, -0.6979) -> (12.4393, 2.2802)
  line L32 (8.4684, 2.7624) -> (12.4393, 2.2802)
  line L33 (26.0668, -0.6979) -> (25.7052, 2.2802)
  line L34 (30.0376, -0.2157) -> (26.0668, -0.6979)
  line L35 (30.0376, -0.2157) -> (29.676, 2.7624)
  line L36 (25.7052, 2.2802) -> (29.676, 2.7624)
  line L37 (43.6203, 3.1321) -> (42.5564, 5.9371)
  line L38 (47.3603, 4.5505) -> (43.6203, 3.1321)
  line L39 (47.3603, 4.5505) -> (46.2965, 7.3555)
  line L40 (42.5564, 5.9371) -> (46.2965, 7.3555)
  line L41 (59.7471, 11.0516) -> (58.0429, 13.5205)
  line L42 (63.039, 13.3238) -> (59.7471, 11.0516)
  line L43 (63.039, 13.3238) -> (61.3348, 15.7928)
  line L44 (58.0429, 13.5205) -> (61.3348, 15.7928)
  line L45 (73.51, 22.6003) -> (71.2645, 24.5897)
  line L46 (76.1625, 25.5944) -> (73.51, 22.6003)
  line L47 (76.1625, 25.5944) -> (73.917, 27.5838)
  line L48 (71.2645, 24.5897) -> (73.917, 27.5838)
  line L49 (84.1093, 37.1072) -> (81.4529, 38.5014)
  line L50 (85.9682, 40.649) -> (84.1093, 37.1072)
  line L51 (85.9682, 40.649) -> (83.3118, 42.0432)
  line L52 (81.4529, 38.5014) -> (83.3118, 42.0432)
  line L53 (90.9288, 53.7291) -> (88.0159, 54.447)
  line L54 (91.886, 57.6129) -> (90.9288, 53.7291)
  line L55 (91.886, 57.6129) -> (88.9732, 58.3308)
  line L56 (88.0159, 54.447) -> (88.9732, 58.3308)
  line L57 (93.5722, 71.5) -> (90.5722, 71.5)
  line L58 (93.5722, 75.5) -> (93.5722, 71.5)
  line L59 (93.5722, 75.5) -> (90.5722, 75.5)
  line L60 (90.5722, 71.5) -> (90.5722, 75.5)
  line L61 (91.886, 89.3871) -> (88.9732, 88.6692)
  line L62 (90.9288, 93.2709) -> (91.886, 89.3871)
  line L63 (90.9288, 93.2709) -> (88.0159, 92.553)
  line L64 (88.9732, 88.6692) -> (88.0159, 92.553)
  line L65 (85.9682, 106.351) -> (83.3118, 104.9568)
  line L66 (84.1093, 109.8928) -> (85.9682, 106.351)
  line L67 (84.1093, 109.8928) -> (81.4529, 108.4986)
  line L68 (83.3118, 104.9568) -> (81.4529, 108.4986)
  line L69 (76.1625, 121.4056) -> (73.917, 119.4162)
  line L70 (73.51, 124.3997) -> (76.1625, 121.4056)
  line L71 (73.51, 124.3997) -> (71.2645, 122.4103)
  line L72 (73.917, 119.4162) -> (71.2645, 122.4103)
  line L73 (63.039, 133.6762) -> (61.3348, 131.2072)
  line L74 (59.7471, 135.9484) -> (63.039, 133.6762)
  line L75 (59.7471, 135.9484) -> (58.0429, 133.4795)
  line L76 (61.3348, 131.2072) -> (58.0429, 133.4795)
  line L77 (47.3603, 142.4495) -> (46.2965, 139.6445)
  line L78 (43.6203, 143.8679) -> (47.3603, 142.4495)
  line L79 (43.6203, 143.8679) -> (42.5564, 141.0629)
  line L80 (46.2965, 139.6445) -> (42.5564, 141.0629)
  line L81 (30.0376, 147.2157) -> (29.676, 144.2376)
  line L82 (26.0668, 147.6979) -> (30.0376, 147.2157)
  line L83 (26.0668, 147.6979) -> (25.7052, 144.7198)
  line L84 (29.676, 144.2376) -> (25.7052, 144.7198)
  line L85 (12.0777, 147.6979) -> (12.4393, 144.7198)
  line L86 (8.1068, 147.2157) -> (12.0777, 147.6979)
  line L87 (8.1068, 147.2157) -> (8.4684, 144.2376)
  line L88 (12.4393, 144.7198) -> (8.4684, 144.2376)
  line L89 (-5.4758, 143.8679) -> (-4.412, 141.0629)
  line L90 (-9.2159, 142.4495) -> (-5.4758, 143.8679)
  line L91 (-9.2159, 142.4495) -> (-8.1521, 139.6445)
  line L92 (-4.412, 141.0629) -> (-8.1521, 139.6445)
  line L93 (-21.6026, 135.9484) -> (-19.8984, 133.4795)
  line L94 (-24.8946, 133.6762) -> (-21.6026, 135.9484)
  line L95 (-24.8946, 133.6762) -> (-23.1904, 131.2072)
  line L96 (-19.8984, 133.4795) -> (-23.1904, 131.2072)
  line L97 (-35.3656, 124.3997) -> (-33.12, 122.4103)
  line L98 (-38.0181, 121.4056) -> (-35.3656, 124.3997)
  line L99 (-38.0181, 121.4056) -> (-35.7725, 119.4162)
  line L100 (-33.12, 122.4103) -> (-35.7725, 119.4162)
  line L101 (-45.9648, 109.8928) -> (-43.3084, 108.4986)
  line L102 (-47.8237, 106.351) -> (-45.9648, 109.8928)
  line L103 (-47.8237, 106.351) -> (-45.1673, 104.9568)
  line L104 (-43.3084, 108.4986) -> (-45.1673, 104.9568)
  line L105 (-52.7843, 93.2709) -> (-49.8715, 92.553)
  line L106 (-53.7416, 89.3871) -> (-52.7843, 93.2709)
  line L107 (-53.7416, 89.3871) -> (-50.8287, 88.6692)
  line L108 (-49.8715, 92.553) -> (-50.8287, 88.6692)
  line L109 (26.3425, 1.65) -> (30.3425, 1.65) projected
  line L110 (26.3425, 4.35) -> (26.3425, 1.65) projected
  line L111 (30.3425, 4.35) -> (26.3425, 4.35) projected
  line L112 (30.3425, 1.65) -> (30.3425, 4.35) projected
  line L113 (11.802, 4.35) -> (7.802, 4.35) projected
  line L114 (7.802, 4.35) -> (7.802, 1.65) projected
  line L115 (7.802, 1.65) -> (11.802, 1.65) projected
  line L116 (11.802, 1.65) -> (11.802, 4.35) projected
  line L117 (11.802, 145.35) -> (7.802, 145.35) projected
  line L118 (7.802, 145.35) -> (7.802, 142.65) projected
  line L119 (7.802, 142.65) -> (11.802, 142.65) projected
  line L120 (11.802, 142.65) -> (11.802, 145.35) projected
  line L121 (26.3425, 145.35) -> (26.3425, 142.65) projected
  line L122 (26.3425, 142.65) -> (30.3425, 142.65) projected
  line L123 (30.3425, 142.65) -> (30.3425, 145.35) projected
  line L124 (30.3425, 145.35) -> (26.3425, 145.35) projected
  line L125 (65.7222, 108.1835) -> (68.4222, 108.1835) projected
  line L126 (65.7222, 112.1835) -> (65.7222, 108.1835) projected
  line L127 (68.4222, 108.1835) -> (68.4222, 112.1835) projected
  line L128 (68.4222, 112.1835) -> (65.7222, 112.1835) projected
  line L129 (65.7222, 87.8165) -> (65.7222, 83.8165) projected
  line L130 (65.7222, 83.8165) -> (68.4222, 83.8165) projected
  line L131 (68.4222, 83.8165) -> (68.4222, 87.8165) projected
  line L132 (68.4222, 87.8165) -> (65.7222, 87.8165) projected
  line L133 (68.4222, 63.1835) -> (65.7222, 63.1835) projected
  line L134 (65.7222, 63.1835) -> (65.7222, 59.1835) projected
  line L135 (65.7222, 59.1835) -> (68.4222, 59.1835) projected
  line L136 (68.4222, 59.1835) -> (68.4222, 63.1835) projected
  line L137 (68.4222, 38.8165) -> (65.7222, 38.8165) projected
  line L138 (65.7222, 38.8165) -> (65.7222, 34.8165) projected
  line L139 (68.4222, 34.8165) -> (68.4222, 38.8165) projected
  line L140 (65.7222, 34.8165) -> (68.4222, 34.8165) projected
  point P0 (11.802, 144.6424)
  point P1 (8.3334, 145.35)
  dimension "d177" = 152
  dimension "d180" = 360
  constraints: 210 end point, 4 collinear, 1 centre point, 1 coincident, 1 concentric, 1 midpoint, 209 other
  measures "d177" diameter of A2
extrude "Extrusion11" cut sketch "Sketch13" against normal blind 3 contours L1 L2 L3 L0 | L9 L12 L11 L10 | L13 L16 L15 L14 | L17 L20 L19 L18 | L21 L24 L23 L22 | L25 L28 L27 L26 | L115 L114 L113 L116 L32 L29 | L29 L32 L116 L115 | L110 L111 L112 L109 L35 L36 | L36 L35 L109 L110 | L37 L40 L39 L38 | L41 L44 L43 L42 | L73 L76 L75 L74 | L77 L80 L79 L78 | L124 L123 L122 L121 L84 L81 | L81 L84 L121 L124 | L120 L119 L118 L117 L87 L88 | L88 L87 L117 L120 | L89 L92 L91 L90 | L93 L96 L95 L94 | L97 L100 L99 L98 | L101 L104 L103 L102 | L105 L108 L107 L106 | L126 L128 L127 L125 | L132 L131 L130 L129 | L136 L135 L134 L133 | L139 L140 L138 L137 bodies 2
body "Solid1"
body "Solid2"
body "Solid3"
